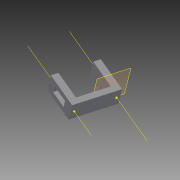
# Autodesk Inventor part: servo_attachement
Saved by Autodesk Inventor 2015 SP1 (Build 190203100, 203)
## iProperties
Created: 2015-07-14
Part Number: servo_attachement
Material: Generic
Document SubType Name: Modeling
Designer: Alexandre Cherpillod
Density: 1 g/cm^3
Appearance: Default
Author: Alexandre Cherpillod
Autodesk Inventor part; units mm, degrees
ref_plane "YZ Plane" through (0, 0, 0) normal (1, 0, 0) x (0, 1, 0)
ref_plane "Work Plane10" through (-7.1266, 5.8946, 10.4647) normal (0.9341198, -0.2351055, -0.2685995) x (-0.2685995, 0.0326501, -0.9626984)
sketch "Sketch2" plane through (-7.1266, 5.8946, 10.4647) normal (0.9341198, -0.2351055, -0.2685995) x (-0.2685995, 0.0326501, -0.9626984)
  line L0 (0, 5) -> (12.2, 5)
  line L1 (12.2, 5) -> (12.2, 0)
  line L2 (12.2, 0) -> (0, 0)
  line L3 (0, 0) -> (0, 5)
  line L4 (12.2, -28) -> (0, -28)
  line L5 (0, -28) -> (0, -23)
  line L6 (0, -23) -> (12.2, -23)
  line L7 (12.2, -23) -> (12.2, -28)
  point P0 (7.9677, -3.709)
  constraints: 16 end point, 4 parallel, 2 horizontal, 2 perpendicular
extrude "Extrusion2" add sketch "Sketch2" along normal blind 20
ref_plane "Work Plane12" through (-19.3217, -20.3191, 0.3055) normal (-0.2351055, -0.9714213, 0.0326501) x (0.9341198, -0.2351055, -0.2685995)
sketch "Sketch4" plane through (-19.3217, -20.3191, 0.3055) normal (-0.2351055, -0.9714213, 0.0326501) x (0.9341198, -0.2351055, -0.2685995)
  line L0 (7.7802, 8.6462) -> (19.9601, 8.6462)
  line L1 (19.9601, 8.6462) -> (19.9601, 3.5538)
  line L2 (19.9601, 3.5538) -> (7.7802, 3.5538)
  line L3 (7.7802, 3.5538) -> (7.7802, 8.6462)
  line L4 (43.7973, 6.1) -> (-30.4435, 6.1) projected
  point P0 (13.3537, 4.2323)
  point P1 (7.7802, 6.1)
  constraints: 8 end point, 2 parallel, 1 horizontal, 1 midpoint, 1 perpendicular, 1 point on line
extrude "Extrusion4" cut sketch "Sketch4" against normal up to surface (5 mm away)
ref_plane "Work Plane11" through (11.5558, 1.1925, 5.0927) normal (0.9341198, -0.2351055, -0.2685995) x (-0.2685995, 0.0326501, -0.9626984)
sketch "Sketch5" plane through (11.5558, 1.1925, 5.0927) normal (0.9341198, -0.2351055, -0.2685995) x (-0.2685995, 0.0326501, -0.9626984)
  line L0 (12.2, 5) -> (0, 5)
  line L1 (0, 5) -> (0, -28)
  line L2 (0, -28) -> (12.2, -28)
  line L3 (12.2, -28) -> (12.2, 5)
  point P0 (7.9677, -3.709)
  constraints: 8 end point, 2 parallel, 1 horizontal, 1 perpendicular
extrude "Extrusion5" add sketch "Sketch5" along normal blind 4.25
hole "Hole1" at (-14.7602, -18.6775, 5.4248) direction (0.9341198, -0.2351055, -0.2685995) diameter 2 depth 8 tip angle 118
hole "Hole3" at (-8.1773, 8.5223, 4.5106) direction (0.9341198, -0.2351055, -0.2685995) diameter 2 depth 8 tip angle 118
thread "Thread1" size "M2x0.4" class "6H" standard "ANSI Metric M Profile" full length
thread "Thread2" size "M2x0.4" class "6H" standard "ANSI Metric M Profile" full length
hole "Hole4" at (7.8922, -24.3788, -1.0887) direction (-0.9341198, 0.2351055, 0.2685995) diameter 2 depth 8 tip angle 118
hole "Hole5" at (14.4752, 2.821, -2.0029) direction (-0.9341198, 0.2351055, 0.2685995) diameter 2 depth 8 tip angle 118
thread "Thread3" size "M2x0.4" class "6H" standard "ANSI Metric M Profile" full length
body "Solid3"
